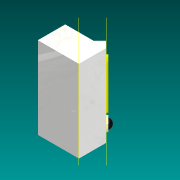
# Autodesk Inventor part: 挂载摄像头
Saved by Autodesk Inventor 2021 (Build 250183000, 183)
## iProperties
Created: 2025-04-18
Part Number: 挂载摄像头
Material: 常规
Document SubType Name: Modeling
Designer: 86155
Density: 1 g/cm^3
Appearance: 默认
Author: 86155
Autodesk Inventor part; units mm, degrees
ref_plane "YZ Plane" through (0, 0, 0) normal (1, 0, 0) x (0, 1, 0)
ref_plane "XZ Plane" through (0, 0, 0) normal (0, 1, 0) x (-1, 0, 0)
ref_plane "XY Plane" through (0, 0, 0) normal (0, 0, 1) x (1, 0, 0)
sketch "草图1" plane through (0, 0, 0) normal (0, 0, 1) x (1, 0, 0)
  line L0 (0, 0) -> (30, 0)
  line L1 (30, 0) -> (30, -60)
  line L2 (30, -60) -> (0, -60)
  line L3 (0, -60) -> (0, 0)
  dimension "d0" = 30
  dimension "d1" = 60
  constraints: 8 end point, 2 parallel, 1 horizontal, 1 perpendicular
  measures "d0" distance of L1.end L2.end
  measures "d1" distance of L0.end L1.end
extrude "拉伸1" add sketch "草图1" along normal blind 20
ref_plane "工作平面2" through (30, -30, 0) normal (-0.7071068, 0, 0.7071068) x (0, -1, 0)
ref_plane "工作平面1" through (30, 0, 20) normal (-0.7071068, 0, 0.7071068) x (0, -1, 0)
sketch "草图2" plane through (30, -30, 0) normal (-0.7071068, 0, 0.7071068) x (0, -1, 0)
  line L0 (25, -5) -> (-25, -5) construction
  line L1 (25, 0) -> (-25, 0)
  line L2 (-25, -10) -> (25, -10)
  arc A0 (25, -10) -> (25, 0) centre (25, -5) ccw
  arc A1 (-25, 0) -> (-25, -10) centre (-25, -5) ccw
  line L3 (30, 0) -> (-30, 0) projected
  point P0 (-30, -21.2132)
  point P1 (0, -5)
  dimension "d4" = 25
  dimension "d5" = 10
  constraints: 8 end point, 4 point on circle, 4 tangent, 2 centre point, 1 collinear, 1 horizontal, 1 midpoint, 1 parallel
  measures "d4" distance of point (0, -5) L0.end
  measures "d5" diameter of A1
extrude "拉伸2" add sketch "草图2" along normal up to surface surface through (15, -30, 0) normal (0, 0, 1)
sketch "草图3" plane through (30, -30, 0) normal (0.7071068, 0, -0.7071068) x (-0.7071068, 0, -0.7071068)
  circle A0 centre (5, -21.4199) radius 3.5
  line L0 (0, -25) -> (0, 25) projected
  line L1 (1.5, -21.4199) -> (8.5, -21.4199)
  point P0 (21.2132, 30)
  dimension "d8" = 7
  dimension "d9" = 5
  constraints: 2 end point, 2 point on circle, 1 centre point, 1 horizontal
  measures "d8" diameter of A0
  measures "d9" distance from line of L0 A0.centre
revolve "旋转1" add sketch "草图3" angle 360 about axis through (28.9393, -51.4199, -1.0607) along (-0.7071068, 0, -0.7071068) picked at (5.8733, -20.6463) contours L1 A0
sketch "草图4" plane through (30, -30, 0) normal (0.7071068, 0, -0.7071068) x (-0.7071068, 0, -0.7071068)
  circle A0 centre (5, -21.4199) radius 3.5 projected
  circle A1 centre (5, -21.4199) radius 4.5
  point P0 (21.2132, 30)
  dimension "d11" = 9
  constraints: 1 centre point, 1 coincident
  measures "d11" diameter of A1
extrude "拉伸3" add sketch "草图4" along normal blind 1 contours A0 | A1
sketch "草图5" plane through (30, -30, 0) normal (0.7071068, 0, -0.7071068) x (-0.7071068, 0, -0.7071068)
  line L0 (5, -11.0678) -> (5, 18.9322) construction
  line L1 (8, -11.0678) -> (8, 18.9322)
  line L2 (2, 18.9322) -> (2, -11.0678)
  arc A0 (2, -11.0678) -> (8, -11.0678) centre (5, -11.0678) ccw
  arc A1 (8, 18.9322) -> (2, 18.9322) centre (5, 18.9322) ccw
  line L3 (0, -25) -> (0, 25) projected
  point P0 (21.2132, 30)
  point P1 (5, 3.9322)
  dimension "d14" = 15
  dimension "d15" = 6
  dimension "d16" = 2
  constraints: 8 end point, 4 point on circle, 4 tangent, 2 centre point, 1 midpoint, 1 parallel, 1 vertical
  measures "d14" distance of point (5, 3.932) L0.end
  measures "d15" diameter of A1
  measures "d16" distance between parallel lines of L3 L2
extrude "拉伸4" add sketch "草图5" along normal blind 1
